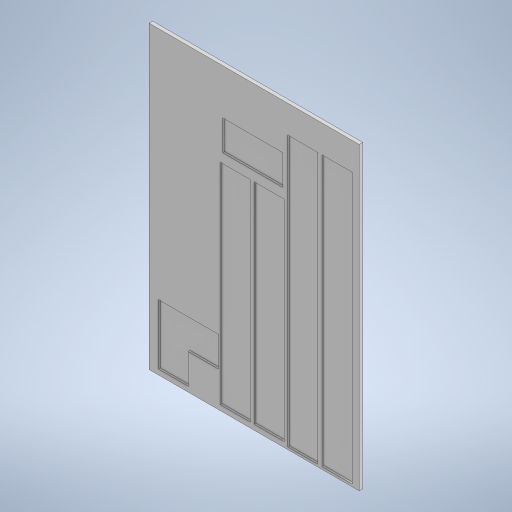
# Autodesk Inventor part: binicial
Saved by Autodesk Inventor 2023 (Build 270158000, 158)
## iProperties
Created: 2022-11-19
Part Number: binicial
Material: Genérico
Document SubType Name: Modeling
Designer: Daniel
Density: 1 g/cm^3
Appearance: Valor por defecto
Author: Daniel
Autodesk Inventor part; units mm, degrees
ref_plane "YZ Plane" through (0, 0, 0) normal (1, 0, 0) x (0, 1, 0)
ref_plane "XZ Plane" through (0, 0, 0) normal (0, 1, 0) x (-1, 0, 0)
ref_plane "XY Plane" through (0, 0, 0) normal (0, 0, 1) x (1, 0, 0)
sketch "Boceto1" plane through (0, 0, 0) normal (0, 0, 1) x (1, 0, 0)
  line L0 (-175, 250) -> (175, 250)
  line L1 (175, 250) -> (175, -250)
  line L2 (175, -250) -> (-175, -250)
  line L3 (-175, -250) -> (-175, 250)
  line L4 (-175, 250) -> (175, -250) construction
  line L5 (175, 250) -> (-175, -250) construction
  point P0 (0, 0)
  dimension "d0" = 350
  dimension "d1" = 500
  constraints: 12 end point, 2 midpoint, 2 parallel, 1 horizontal, 1 perpendicular
  measures "d0" distance of L1.end L2.end
  measures "d1" distance of L0.end L1.end
extrude "Extrusión1" add sketch "Boceto1" along normal blind 6
sketch "Boceto2" plane through (0, 0, 6) normal (0, 0, 1) x (1, 0, 0)
  line L0 (-175, -250) -> (175, -250) projected
  line L1 (-175, -250) -> (-159.7, -250)
  line L2 (-159.7, -250) -> (-159.7, -241.31)
  line L3 (-159.7, -241.31) -> (-175, -241.31)
  line L4 (-175, -241.31) -> (-175, -250)
  line L5 (-159.7, -241.31) -> (-159.7, -141.31)
  line L6 (-159.7, -141.31) -> (-59.7, -141.31)
  line L7 (-59.7, -141.31) -> (-59.7, -191.31)
  line L8 (-59.7, -191.31) -> (-109.7, -191.31)
  line L9 (-159.7, -241.31) -> (-109.7, -241.31)
  line L10 (-109.7, -241.31) -> (-109.7, -191.31)
  line L11 (-109.7, -241.31) -> (-56.7, -241.31)
  line L12 (-56.7, -241.31) -> (-6.7, -241.31)
  line L13 (-6.7, -241.31) -> (-6.7, 108.59)
  line L14 (-6.7, 108.59) -> (-56.7, 108.59)
  line L15 (-56.7, 108.59) -> (-56.7, -241.31)
  line L16 (-6.7, -241.31) -> (-0.14, -241.31)
  line L17 (-0.14, -241.31) -> (49.86, -241.31)
  line L18 (49.86, -241.31) -> (49.86, 108.59)
  line L19 (49.86, 108.59) -> (-0.14, 108.59)
  line L20 (-0.14, 108.59) -> (-0.14, -241.31)
  line L21 (49.86, -241.31) -> (55.86, -241.31)
  line L22 (55.86, -241.31) -> (55.86, -245.92)
  line L23 (55.86, -245.92) -> (49.86, -245.92)
  line L24 (49.86, -245.92) -> (49.86, -241.31)
  line L25 (55.86, -245.92) -> (105.86, -245.92)
  line L26 (105.86, -245.92) -> (105.86, 204.08)
  line L27 (105.86, 204.08) -> (55.86, 204.08)
  line L28 (55.86, 204.08) -> (55.86, -245.92)
  line L29 (105.86, -245.92) -> (113.01, -245.92)
  line L30 (113.01, -245.92) -> (163.01, -245.92)
  line L31 (163.01, -245.92) -> (163.01, 204.08)
  line L32 (163.01, 204.08) -> (113.01, 204.08)
  line L33 (113.01, 204.08) -> (113.01, -245.92)
  line L34 (49.86, 108.59) -> (47.86, 108.59)
  line L35 (47.86, 108.59) -> (47.86, 124.59)
  line L36 (47.86, 124.59) -> (49.86, 124.59)
  line L37 (49.86, 124.59) -> (49.86, 108.59)
  line L38 (47.86, 124.59) -> (-52.14, 124.59)
  line L39 (-52.14, 124.59) -> (-52.14, 174.59)
  line L40 (-52.14, 174.59) -> (47.86, 174.59)
  line L41 (47.86, 174.59) -> (47.86, 124.59)
  point P0 (0, 0)
  dimension "d4" = 15.3
  dimension "d5" = 8.69
  dimension "d6" = 100
  dimension "d7" = 100
  dimension "d8" = 50
  dimension "d9" = 50
  dimension "d10" = 53
  dimension "d11" = 50
  dimension "d12" = 349.9
  dimension "d13" = 6.56
  dimension "d14" = 50
  dimension "d15" = 349.9
  dimension "d16" = 6
  dimension "d17" = 4.61
  dimension "d18" = 50
  dimension "d19" = 450
  dimension "d20" = 7.15
  dimension "d21" = 50
  dimension "d22" = 450
  dimension "d23" = 2
  dimension "d24" = 16
  dimension "d25" = 100
  dimension "d26" = 50
  constraints: 82 end point, 16 parallel, 12 horizontal, 10 perpendicular, 2 vertical, 1 point on line
  measures "d4" distance of L3.end L2.end
  measures "d5" distance of L1.end L2.end
  measures "d6" distance of L2.end L5.end
  measures "d7" distance of L5.end L6.end
  measures "d8" distance of L6.end L7.end
  measures "d9" distance of L7.end L8.end
  measures "d10" distance of L9.end L11.end
  measures "d11" distance of L14.end L13.end
  measures "d12" distance of L13.end L12.end
  measures "d13" distance of L12.end L16.end
  measures "d14" distance of L19.end L18.end
  measures "d15" distance of L18.end L17.end
  measures "d16" distance of L22.end L23.end
  measures "d17" distance of L21.end L22.end
  measures "d18" distance of L27.end L26.end
  measures "d19" distance of L26.end L25.end
  measures "d20" distance of L25.end L29.end
  measures "d21" distance of L32.end L31.end
  measures "d22" distance of L31.end L30.end
  measures "d23" distance of L35.end L36.end
  measures "d24" distance of L34.end L35.end
  measures "d25" distance of L39.end L40.end
  measures "d26" distance of L38.end L39.end
extrude "Extrusión2" cut sketch "Boceto2" against normal blind 3 contours L38 L39 L40 L41 | L33 L32 L31 L30 | L20 L19 L18 L17 | L15 L14 L13 L12 | L5 L6 L7 L8 L10 L9 | L28 L27 L26 L25 L22
